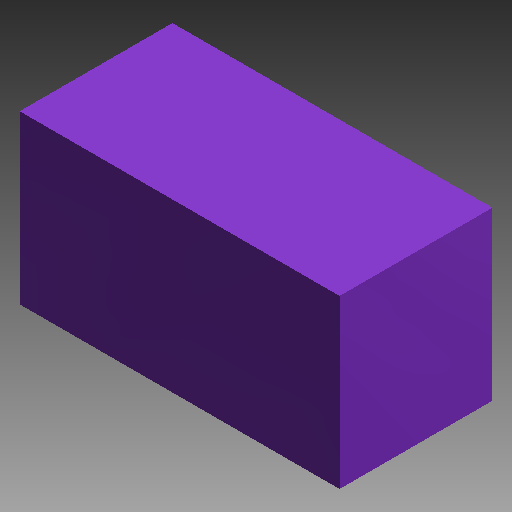
# Autodesk Inventor part: 4.7uF
Saved by Autodesk Inventor 2018.2 (Build 222227000, 227)
## iProperties
Part Number: 4.7uF
Material: Generic
Document SubType Name: Modeling
Designer: autocad
Appearance: C1206, 4.7uF
Author: autocad
Autodesk Inventor part; units mm, degrees
ref_plane "YZ Plane" through (0, 0, 0) normal (1, 0, 0) x (0, 1, 0)
ref_plane "XZ Plane" through (0, 0, 0) normal (0, 1, 0) x (-1, 0, 0)
ref_plane "XY Plane" through (0, 0, 0) normal (0, 0, 1) x (1, 0, 0)
sketch "C1206, 4.7uF_71" plane through (0, 0, 0) normal (0, 0, 1) x (1, 0, 0)
  line L0 (-1.675, 0.875) -> (1.675, 0.875)
  line L1 (1.675, 0.875) -> (1.675, -0.875)
  line L2 (1.675, -0.875) -> (-1.675, -0.875)
  line L3 (-1.675, -0.875) -> (-1.675, 0.875)
  constraints: 8 end point
extrude "Extrusion1" add sketch "C1206, 4.7uF_71" along normal blind 1.6
body "Solid1"
